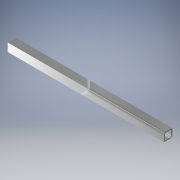
# Autodesk Inventor part: 15102898-16-P-0307
Saved by Autodesk Inventor 2017 (Build 210142000, 142)
## iProperties
Created: 2016-10-08
Part Number: 15102898-16-P-0307
Material: Aluminum 6061
Document SubType Name: Modeling
Designer: gus
Density: 2.7 g/cm^3
Appearance: Aluminum - Flat
Author: gus
Autodesk Inventor part; units mm, degrees
ref_plane "YZ Plane" through (0, 0, 0) normal (1, 0, 0) x (0, 1, 0)
ref_plane "XZ Plane" through (0, 0, 0) normal (0, 1, 0) x (-1, 0, 0)
ref_plane "XY Plane" through (0, 0, 0) normal (0, 0, 1) x (1, 0, 0)
sketch "Sketch1" plane through (0, 0, 0) normal (1, 0, 0) x (0, 1, 0)
  line L0 (0, 0) -> (-25.4, 0)
  line L1 (-25.4, 0) -> (-25.4, -25.4)
  line L2 (-25.4, -25.4) -> (0, -25.4)
  line L3 (0, -25.4) -> (0, 0)
  line L4 (-3.175, -22.225) -> (-22.225, -22.225)
  line L5 (-22.225, -22.225) -> (-22.225, -3.175)
  line L6 (-22.225, -3.175) -> (-3.175, -3.175)
  line L7 (-3.175, -3.175) -> (-3.175, -22.225)
  dimension "d0" = 25.4
  dimension "d1" = 25.4
  dimension "d2" = 3.175
  constraints: 16 end point, 4 parallel, 2 perpendicular, 1 horizontal, 3 other
  measures "d0" distance of L2.end L1.end
  measures "d1" distance of L1.end L0.end
  measures "d2" distance between parallel lines of L2 L4
extrude "Extrusion1" add sketch "Sketch1" along normal blind 482.6
sketch "Sketch2" plane through (0, 0, 0) normal (0, 1, 0) x (1, 0, 0)
  line L0 (0, 3.175) -> (0, 22.225) projected
  line L1 (0, 12.7) -> (482.6, 12.7) construction
  line L2 (0, 25.4) -> (482.6, 25.4) projected
  line L3 (482.6, 25.4) -> (482.6, 0) projected
  point P0 (0, 0)
  point P1 (444.5, 12.7)
  point P2 (12.7, 12.7)
  point P3 (38.1, 12.7)
  point P4 (465.6836, 11.7602)
  dimension "d6" = 12.7
  dimension "d7" = 12.7
  dimension "d8" = 38.1
  dimension "d9" = 38.1
  dimension "d10" = 16.9164
  dimension "d11" = 13.6398
  constraints: 3 point on line, 2 end point, 2 midpoint
  measures "d6" distance of L2.end L1.end
  measures "d7" distance from line of L0 point (12.7, 12.7)
  measures "d8" distance from line of L0 point (38.1, 12.7)
  measures "d9" distance from line of L3 point (444.5, 12.7)
  measures "d10" distance from line of L3 point (465.684, 11.76)
  measures "d11" distance from line of L2 point (465.684, 11.76)
hole "Hole1" at (444.5, 0, -12.7) at (12.7, 0, -12.7) at (38.1, 0, -12.7) at (465.6836, 0, -11.7602) direction (0, -1, 0) diameter 6.35 end through all
body "Solid1"
